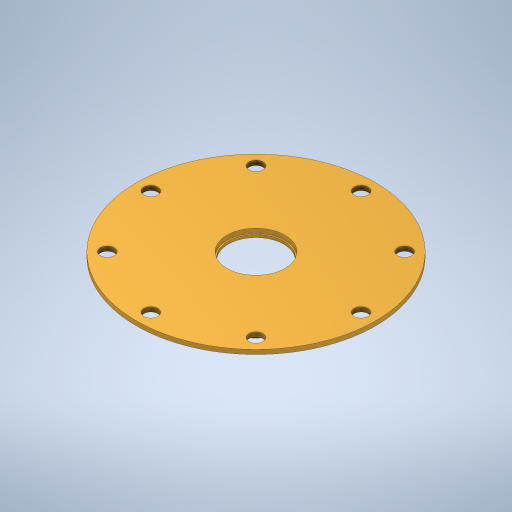
# Autodesk Inventor part: Flange
Saved by Autodesk Inventor 2024 (Build 280153000, 153)
## iProperties
Created: 2023-10-26
Part Number: Flange
Material: Brass, Soft Yellow
Document SubType Name: Modeling
Designer: schanen
Density: 8.47 g/cm^3
Appearance: Brass - Satin
Author: schanen
Autodesk Inventor part; units mm, degrees
ref_plane "YZ Plane" through (0, 0, 0) normal (1, 0, 0) x (0, 1, 0)
ref_plane "XZ Plane" through (0, 0, 0) normal (0, 1, 0) x (-1, 0, 0)
ref_plane "XY Plane" through (0, 0, 0) normal (0, 0, 1) x (1, 0, 0)
sketch "Sketch2" plane through (0, 0, 0) normal (0, 0, 1) x (1, 0, 0)
  line L0 (-82.5, 0) -> (-82.5, 2.5)
  line L1 (-82.5, 2.5) -> (-103.5, 2.5)
  line L2 (-103.5, 2.5) -> (-103.5, 6.35)
  line L3 (-103.5, 6.35) -> (-25, 6.35)
  line L4 (-25, 6.35) -> (-25, 2.35)
  line L5 (-25, 2.35) -> (-24, 2.35)
  line L6 (-24, 2.35) -> (-24, 0)
  line L7 (-24, 0) -> (-82.5, 0)
  line L8 (0, -1.27) -> (0, 7.62) projected
  point P0 (0, 0)
  dimension "d1" = 103.5
  dimension "d2" = 6.35
  dimension "d3" = 2.5
  dimension "d4" = 82.5
  dimension "d5" = 4
  dimension "d6" = 25
  dimension "d7" = 1
  constraints: 16 end point, 5 perpendicular, 1 horizontal, 1 horizontal alignment, 1 vertical
  measures "d1" distance from line of point (0, 0) L2
  measures "d2" distance between parallel lines of L7 L3
  measures "d3" distance between parallel lines of L7 L1
  measures "d4" distance from line of point (0, 0) L0
  measures "d5" distance between parallel lines of L3 L5
  measures "d6" distance from line of point (0, 0) L4
  measures "d7" distance of L4.end L5.end
revolve "Revolution1" add sketch "Sketch2" angle 360 about axis through (0, -10, 0) along (0, 1, 0)
sketch "Sketch3" plane through (0, 6.35, 0) normal (0, 1, 0) x (1, 0, 0)
  point P0 (0, 0)
  point P1 (0, 91)
  dimension "d10" = 91
  measures "d10" distance of point (0, 0) point (0, 91)
hole "Hole1" at (0, 6.35, -91) direction (0, -1, 0) diameter 12 end through all
pattern_circular "Circular Pattern1" count 8 over 360 about axis through (0, 4.425, 0) along (0, 1, 0) of "Hole1"
sketch "Sketch4" plane through (0, 0, 0) normal (0, -1, 0) x (1, 0, 0)
  point P0 (0, 0)
  point P1 (55, 0)
  dimension "d21" = 55
  constraints: 1 horizontal alignment
  measures "d21" distance of point (55, 0) point (0, 0)
hole "Hole2" at (55, 0, 0) direction (0, 1, 0) diameter 3.242 depth 4 tip angle 118 thread size "M4x0.7" class "6H" standard "ISO Metric profile"
pattern_circular "Circular Pattern2" count 3 over 360 about axis through (0, 1.175, 0) along (0, 1, 0) of "Hole2"
body "Solid1"
